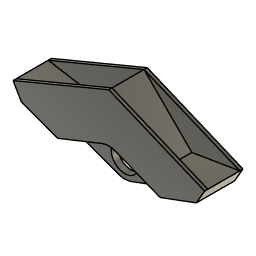
pool (Autodesk Fusion 360 design; units mm, degrees)
Autodesk Fusion 360 part; units mm, degrees
note: some values were not read from the file. Set by a fixed rule: which face or edge a step refers to.
sketch "Sketch1" plane through (0, 0, 0) normal (0, 1, 0) x (1, 0, 0)
  line L0 (-30, 0) -> (0, -30)
  line L1 (0, 0) -> (-30, 0)
  line L2 (0, 0) -> (0, -55)
  line L3 (-30, 0) -> (-60, -5)
  circle A0 centre (0, 12) radius 4.5
  circle A1 centre (0, 12) radius 8.55
  line L4 (-60, -5) -> (-54.8038, 4)
  line L5 (-60, -5) -> (-60.4903, -5) construction
  line L6 (-54.8038, 4) -> (-3.9877, 22.7865)
  line L7 (60, -5) -> (54.8038, 4)
  line L8 (30, 0) -> (60, -5)
  line L9 (30, 0) -> (0, -30)
  line L10 (-60, -5) -> (0, -30)
  line L11 (60, -5) -> (0, -30)
  circle A2 centre (0, 12) radius 11.5
  line L12 (-32.1229, 12.385) -> (-4.2451, 1.3122)
  line L13 (32.1229, 12.385) -> (4.2451, 1.3122)
  line L14 (54.8038, 4) -> (3.9877, 22.7865)
  dimension "d3" = 30
  dimension "d4" = 30
  dimension "d6" = 30
  dimension "d7" = 5
  dimension "d8" = 9
  dimension "d9" = 17.1
  dimension "d10" = 60
  dimension "d11" = 12
  dimension "d12" = 23
  dimension "d31" = 4
  constraint coincident L1.start L2.start
  constraint horizontal L1
  constraint perpendicular L1 L2
  constraint coincident L0.end L2
  constraint concentric A0 A1
  constraint horizontal L5
  constraint symmetric L0.start L2 L8.start
  constraint symmetric L0.end L2 L9.end
  constraint symmetric L2 L3.end L7.start
  constraint symmetric L2 L7.end L4.end
  constraint coincident L2 A0.centre
  constraint symmetric L2 L0.end L9.end
  constraint concentric A0 A2
  constraint tangent L6 A2
  constraint coincident L6.end A2
  constraint coincident L6 L12.start
  constraint coincident A2 L12.end
  constraint tangent A2 L12
  constraint symmetric L2 L6.end L14.end
  constraint symmetric L2 L12.start L13.start
  constraint symmetric L2 L12.end L13.end
  constraint symmetric L2 L4.end L7.end
  measures "d3" distance of L1.start L0.end
  measures "d4" distance of L1.start L0.start
  measures "d6" horizontal distance of L0.start L3.end
  measures "d7" vertical distance of L0.start L3.end
  measures "d8" diameter of A0
  measures "d9" diameter of A1
  measures "d10" angle of L4 L5
  measures "d11" distance of L1.start A0.centre
  measures "d12" diameter of A2
  measures "d31" vertical distance of L0.start L4.end
extrude "Extrude1" add sketch "Sketch1" along normal mid plane 24 contours L0 L1 L2 | L1 L2 L3 L4 L6 L7 L8 L9 A2 L12 L13 L14 | L0 L3 L10 | L8 L9 L11
extrude "Extrude2" cut sketch "Sketch1" along normal mid plane 20 contours L0 L3 L10 | L8 L9 L11
extrude "Extrude3" add sketch "Sketch1" along normal mid plane 4 contours L6 A2 L12 | A2 L13 L14 | A2
sketch "Sketch2" plane through (-7.8906, 0, -21.3436) normal (-0.346757, 0, -0.937955) x (0, -1, 0)
  line L0 (2, 25.8353) -> (12, 25.8353)
  line L1 (12, 25.8353) -> (12, 50.0165)
  line L2 (12, 50.0165) -> (-12, 50.0165)
  line L3 (-12, 50.0165) -> (-12, 25.8353)
  line L4 (-12, 25.8353) -> (-2, 25.8353)
  line L5 (-2, 25.8353) -> (-2, -4.1611)
  line L6 (-2, -4.1611) -> (2, -4.1611)
  line L7 (2, -4.1611) -> (2, 25.8353)
  circle A0 centre (0, 33.8389) radius 5
  circle A1 centre (0, 33.8389) radius 7
  circle A2 centre (0, 42.8389) radius 2.05
  circle A3 centre (0, 24.8389) radius 2.05
  circle A4 centre (0, 42.8389) radius 3
  circle A5 centre (0, 24.8389) radius 3
  dimension "d19" = 10
  dimension "d20" = 14
  dimension "d21" = 4.1
  dimension "d22" = 9
  dimension "d23" = 4.1
  dimension "d24" = 9
  dimension "d25" = 6
  dimension "d26" = 6
  dimension "d40" = 38
  constraint concentric A0 A1
  constraint concentric A2 A4
  constraint concentric A3 A5
  measures "d19" diameter of A0
  measures "d20" diameter of A1
  measures "d21" diameter of A2
  measures "d22" distance of A0.centre A2.centre
  measures "d23" diameter of A3
  measures "d24" distance of A0.centre A3.centre
  measures "d25" diameter of A4
  measures "d26" diameter of A5
  measures "d40" distance of L6 A0.centre
extrude "Extrude6" add sketch "Sketch2" along normal up to surface contours L0 L7 A3 A5 | L7 A3 | L5 A3 | L4 L5 A3 A5 end surface through (-32.1229, 0, -12.385) normal (0.369139, 0, -0.929374) offset 0
extrude "Extrude11" cut sketch "Sketch2" against normal blind 7 contours L7 A3 | L5 L7 A1 A3 | A1 A3 | L5 A3 | A1 A2 | A1 A2
sketch "Sketch4" plane through (7.8906, 0, -21.3436) normal (0.346757, 0, -0.937955) x (0, 1, 0)
  line L0 (12, 50.0165) -> (-12, 50.0165)
  line L1 (-12, 50.0165) -> (-12, 25.8353)
  line L2 (-12, 25.8353) -> (-2, 25.8353)
  line L3 (-2, 25.8353) -> (-2, -4.1611)
  line L4 (-2, -4.1611) -> (2, -4.1611)
  line L5 (2, -4.1611) -> (2, 25.8353)
  line L6 (2, 25.8353) -> (12, 25.8353)
  line L7 (12, 25.8353) -> (12, 50.0165)
  circle A0 centre (0, 33.8389) radius 5
  circle A1 centre (0, 33.8389) radius 7
  circle A2 centre (0, 24.8389) radius 2.05
  circle A3 centre (0, 24.8389) radius 3
  circle A4 centre (0, 42.8389) radius 2.05
  circle A5 centre (0, 42.8389) radius 3
  dimension "d44" = 10
  dimension "d45" = 14
  dimension "d46" = 4.1
  dimension "d47" = 6
  dimension "d48" = 9
  dimension "d49" = 4.1
  dimension "d50" = 6
  dimension "d51" = 9
  dimension "d59" = 38
  constraint concentric A0 A1
  constraint concentric A2 A3
  constraint concentric A4 A5
  measures "d44" diameter of A0
  measures "d45" diameter of A1
  measures "d46" diameter of A2
  measures "d47" diameter of A3
  measures "d48" distance of A0.centre A2.centre
  measures "d49" diameter of A4
  measures "d50" diameter of A5
  measures "d51" distance of A0.centre A4.centre
  measures "d59" distance of L4 A0.centre
extrude "Extrude8" add sketch "Sketch4" along normal up to surface contours L5 L6 A2 A3 | L2 L3 A2 A3 | L5 A2 | L3 A2 end surface through (32.1229, 0, -12.385) normal (-0.369139, 0, -0.929374) offset 0
extrude "Extrude10" cut sketch "Sketch4" against normal blind 7 contours L5 A2 | L3 L5 A1 A2 | A1 A2 | L3 A2 | A1 A4 | A1 A4
